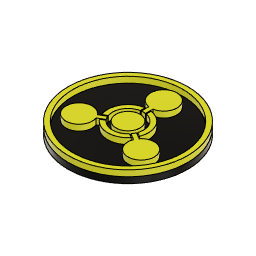
chemicalSymbol (Autodesk Fusion 360 design; units mm, degrees)
Autodesk Fusion 360 part; units mm, degrees
sketch "Sketch1" plane through (0, 0, 0) normal (0, 0, 1) x (1, 0, 0)
  circle A0 centre (0, 0) radius 25
  dimension "d1" = 50
  constraint coincident A0.centre origin
  measures "d1" diameter of A0
extrude "Extrude1" add sketch "Sketch1" along normal blind 2.5 makes body 1
sketch "Sketch2" plane through (0, 0, 2.5) normal (0, 0, 1) x (-1, 0, 0)
  circle A0 centre (0, 0) radius 25
  circle A1 centre (0, 0) radius 5
  circle A2 centre (0, 0) radius 23
  circle A3 centre (0, 0) radius 6.5
  circle A4 centre (0, 0) radius 8.5
  line L0 (0, 0) -> (0, -15) construction
  circle A5 centre (0, -15) radius 5.5
  circle A6 centre (-12.9904, 7.5) radius 5.5
  circle A7 centre (12.9904, 7.5) radius 5.5
  line L1 (-12.9904, 7.5) -> (0, -15) construction
  line L2 (-12.9904, 7.5) -> (12.9904, 7.5) construction
  line L3 (12.9904, 7.5) -> (0, -15) construction
  line L4 (0, 0) -> (-12.9904, 7.5) construction
  line L5 (0, 0) -> (12.9904, 7.5) construction
  line L6 (-0.875, -6.4408) -> (-0.875, -9.57)
  line L7 (0.875, -6.4408) -> (0.875, -9.57)
  line L8 (-1.25, -6.3787) -> (-1.25, -8.4076)
  line L9 (1.25, -6.3787) -> (1.25, -8.4076)
  line L10 (-1.25, -8.4076) -> (1.25, -8.4076) construction
  line L11 (-0.875, -9.57) -> (0.875, -9.57) construction
  line L12 (-7.8504, 5.5428) -> (-5.1404, 3.9782)
  line L13 (-8.7254, 4.0273) -> (-6.0154, 2.4626)
  line L14 (-8.7254, 4.0273) -> (-7.8504, 5.5428) construction
  line L15 (-6.6562, 5.2863) -> (-4.8991, 4.2719)
  line L16 (-7.9062, 3.1213) -> (-6.1491, 2.1068)
  line L17 (-6.6562, 5.2863) -> (-7.9062, 3.1213) construction
  line L18 (5.1404, 3.9782) -> (7.8504, 5.5428)
  line L19 (6.0154, 2.4626) -> (8.7254, 4.0273)
  line L20 (7.8504, 5.5428) -> (8.7254, 4.0273) construction
  line L21 (6.6562, 5.2863) -> (4.8991, 4.2719)
  line L22 (7.9062, 3.1213) -> (6.1491, 2.1068)
  line L23 (6.6562, 5.2863) -> (7.9062, 3.1213) construction
  dimension "d4" = 10
  dimension "d5" = 18
  dimension "d6" = 1.5
  dimension "d7" = 3.5
  dimension "d8" = 11
  dimension "d9" = 15
  dimension "d10" = 1.75
  dimension "d11" = 2.5
  constraint coincident A0.centre A1.centre
  constraint vertical L0
  constraint coincident L0.end A5.centre
  constraint equal A5 A6
  constraint equal A5 A7
  constraint coincident A6.centre L1.start
  constraint coincident A7.centre L2.end
  constraint equal L1 L2
  constraint equal L1 L3
  constraint horizontal L2
  constraint equal L0 L4
  constraint coincident A3 L6.start
  constraint coincident A5 L6.end
  constraint parallel L0 L6
  constraint coincident A3 L7.start
  constraint coincident A5 L7.end
  constraint parallel L6 L7
  constraint coincident A3 L8.start
  constraint coincident A4 L8.end
  constraint vertical L8
  constraint coincident A3 L9.start
  constraint coincident A4 L9.end
  constraint parallel L8 L9
  constraint horizontal L10
  constraint perpendicular L7 L11
  constraint coincident A6 L12.start
  constraint coincident A3 L12.end
  constraint coincident A6 L13.start
  constraint coincident A3 L13.end
  constraint equal L11 L14
  constraint parallel L12 L13
  constraint equal L12 L13
  constraint perpendicular L4 L14
  constraint coincident A4 L15.start
  constraint coincident A3 L15.end
  constraint coincident A4 L16.start
  constraint coincident A3 L16.end
  constraint equal L15 L16
  constraint perpendicular L4 L17
  constraint parallel L15 L16
  constraint equal L10 L17
  constraint coincident A3 L18.start
  constraint coincident A7 L18.end
  constraint coincident A3 L19.start
  constraint coincident A7 L19.end
  constraint perpendicular L5 L20
  constraint equal L18 L19
  constraint parallel L18 L19
  constraint coincident A4 L21.start
  constraint coincident A3 L21.end
  constraint coincident A4 L22.start
  constraint coincident A3 L22.end
  constraint equal L11 L20
  constraint equal L21 L22
  constraint parallel L21 L22
  constraint perpendicular L5 L23
  constraint equal L10 L23
  measures "d4" diameter of A1
  measures "d8" diameter of A5
  measures "d9" distance of A0.centre L0.end
  measures "d10" distance of L6.end L7.end
  measures "d11" distance of L8.end L9.end
extrude "Extrude2" add sketch "Sketch2" along normal blind 2.5 separate body contours A0 | A1 | A3 A4 L9 L22 | A3 A4 L18 L19 | A3 A4 L6 L7 | A4 A7 L18 L19 | A4 A5 L6 L7 | A3 A4 L15 L21 | A7 | A3 A4 L8 L16 | A5 | A3 A4 L12 L13 | A4 A6 L12 L13 | A6 makes body 2 at (5.4586, 6.5156, 4.1667) makes body 3 at (14.9383, -9.9075, 2.5) makes body 4 at (-14.4858, -7.6434, 2.5) makes body 5 at (-5.8824, 6.1358, 4.1667) makes body 6 at (1.8525, 15.362, 2.5) makes body 7 at (-24.9689, 1.2461, 4.1667) makes body 8 at (-4.9938, 0.2492, 4.1667) makes body 9 at (6.3838, -5.6122, 4.1667)
